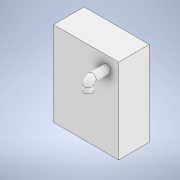
# Autodesk Inventor part: Sump_1SDB_Tub
Saved by Autodesk Inventor 2022 (Build 260153000, 153)
## iProperties
Created: 2021-06-29
Part Number: Sump_1SDB_Tub
Material: Generic
Document SubType Name: Modeling
Designer: jamieson-bl
Density: 1 g/cm^3
Appearance: Default
Author: jamieson-bl
Autodesk Inventor part; units mm, degrees
ref_plane "YZ Plane" through (0, 0, 0) normal (1, 0, 0) x (0, 1, 0)
sketch "Sketch1" plane through (0, 0, 0) normal (0, 0, 1) x (1, 0, 0)
  line L0 (215.9, -280.9875) -> (-215.9, -280.9875)
  line L1 (-215.9, -280.9875) -> (-215.9, 280.9875)
  line L2 (-215.9, 280.9875) -> (215.9, 280.9875)
  line L3 (215.9, 280.9875) -> (215.9, -280.9875)
  line L4 (215.9, -280.9875) -> (-215.9, 280.9875) construction
  line L5 (-215.9, -280.9875) -> (215.9, 280.9875) construction
  point P0 (0, 0)
  dimension "d0" = 431.8
  dimension "d1" = 561.975
  constraints: 12 end point, 2 midpoint, 2 parallel, 1 horizontal, 1 perpendicular
  measures "d0" distance of L1.end L2.end
  measures "d1" distance of L0.end L1.end
extrude "Extrusion1" add sketch "Sketch1" along normal blind 203.2
sketch "Sketch2" plane through (0, 0, 203.2) normal (0, 0, 1) x (1, 0, 0)
  circle A0 centre (139.7, 205.5749) radius 25.4
  line L0 (-215.9, -280.9875) -> (215.9, -280.9875) projected
  line L1 (215.9, -280.9875) -> (215.9, 280.9875) projected
  point P0 (0, 0)
  dimension "d4" = 50.8
  dimension "d5" = 486.5624
  dimension "d6" = 76.2
  constraints: 1 centre point
  measures "d4" diameter of A0
  measures "d5" distance from line of L0 A0.centre
  measures "d6" distance from line of L1 A0.centre
extrude "Extrusion2" add sketch "Sketch2" along normal blind 98.044
ref_plane "Work Plane1" through (-215.9, 177.6349, 0) normal (0, 1, 0) x (1, 0, 0)
sketch "Sketch3" plane through (-215.9, 177.6349, 0) normal (0, 1, 0) x (1, 0, 0)
  circle A0 centre (355.6, -329.184) radius 25.4
  line L0 (330.2, -301.244) -> (381, -301.244) projected
  point P0 (215.9, 0)
  dimension "d16" = 27.94
  constraints: 1 centre point
  measures "d16" distance from line of L0 A0.centre
extrude "Extrusion3" add sketch "Sketch3" against normal blind 36.83
ref_plane "Work Plane2" through (139.7, -280.9875, 0) normal (1, 0, 0) x (0, 0, -1)
sketch "Sketch5" plane through (0, 0, 301.244) normal (0, 0, 1) x (1, 0, 0)
  circle A0 centre (139.7, 205.5749) radius 25.4 projected
  circle A1 centre (139.7, 205.5749) radius 25.4
  line L0 (165.1, 177.6349) -> (114.3, 177.6349) projected
  line L1 (114.3, 177.6349) -> (165.1, 177.6349)
  point P0 (0, 0)
  constraints: 2 end point, 1 centre point, 1 coincident, 1 collinear
revolve "Revolution1" add sketch "Sketch5" angle 90 about axis through (165.1, 177.6349, 301.244) along (1, 0, 0)
body "Solid1"
